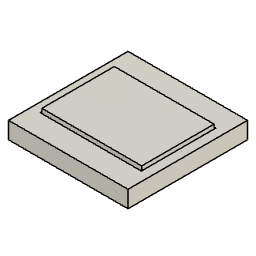
EU_switch (Autodesk Fusion 360 design; units mm, degrees)
Autodesk Fusion 360 part; units mm, degrees
note: some values were not read from the file. Set by a fixed rule: which sketch regions a step uses.
box "BoxPrimitive3" add length 85 width 85 height 12 placed x (0, 1, 0) y (-1, 0, 0) z (0, 0, 1) at (85, 0, 0) makes body 1 in component "panel"
ref_plane "WorkPlane1" through (42.5, 42.5, 12) normal (0, 0, 1) x (0, 1, 0) in component "panel"
sketch "Sketch5" plane through (42.5, 42.5, 12) normal (0, 0, 1) x (1, 0, 0) in component "panel"
  line L0 (-36, 26.5) -> (36, 26.5)
  line L1 (36, 26.5) -> (36, -26.5)
  line L2 (36, -26.5) -> (-36, -26.5)
  line L3 (-36, -26.5) -> (-36, 26.5)
  dimension "d59" = 72
  dimension "d60" = 53
  dimension "d61" = 36
  dimension "d63" = 26.5
  constraint horizontal L0
  constraint vertical L1
  constraint horizontal L2
  constraint vertical L3
  measures "d59" distance of L0.start L0.end
  measures "d60" distance of L0.start L2.end
  measures "d61" distance of origin L1
  measures "d63" distance of origin L0
extrude "Extrude3" cut sketch "Sketch5" against normal through all bodies 1 in component "panel"
ref_plane "WorkPlane2" through (42.5, 42.5, 0) normal (0, 0, -1) x (0, -1, 0) in component "panel"
sketch "Sketch7" plane through (42.5, 42.5, 0) normal (0, 0, -1) x (1, 0, 0) in component "panel"
  line L0 (-40, 40) -> (40, 40)
  line L1 (40, 40) -> (40, -40)
  line L2 (40, -40) -> (-40, -40)
  line L3 (-40, -40) -> (-40, 40)
  line L4 (-42.5, 42.5) -> (-42.5, -42.5)
  line L5 (42.5, -42.5) -> (42.5, 42.5)
  line L6 (42.5, 42.5) -> (-42.5, 42.5)
  line L7 (-42.5, -42.5) -> (42.5, -42.5)
  dimension "d110" = 2.5
  dimension "d112" = 2.5
  dimension "d113" = 2.5
  dimension "d114" = 2.5
  constraint horizontal L0
  constraint vertical L1
  constraint horizontal L2
  constraint vertical L3
  measures "d110" distance of L0.start L4
  measures "d112" distance of L0.end L5
  measures "d113" distance of L0.start L6
  measures "d114" distance of L2.end L7
extrude "Extrude4" cut sketch "Sketch7" against normal blind 10 contours L0 L1 L2 L3 bodies 1 in component "panel"
ref_plane "WorkPlane1" through (42.5, 42.5, 11) normal (-1, 0, 0) x (0, 1, 0) in component "Button"
sketch "Sketch3" plane through (42.5, 42.5, 11) normal (-1, 0, 0) x (0, 1, 0) in component "Button"
  line L0 (-25.7589, 3.5328) -> (-25.7589, -3.5328)
  line L1 (-25.7589, -3.5328) -> (25.7589, -3.5328)
  line L2 (25.7589, -3.5328) -> (25.7589, 3.5328)
  line L3 (25.7589, 3.5328) -> (-25.7589, 3.5328)
  line L4 (-25.7589, 3.5328) -> (25.7589, -3.5328) construction
  line L5 (-25.7589, -3.5328) -> (25.7589, 3.5328) construction
  line L6 (-25.7589, -3.5328) -> (-24.8077, 3.4023) construction
  line L7 (25.7589, -3.5328) -> (24.8077, 3.4023) construction
  line L8 (0, 0) -> (0, -3.5328) construction
  dimension "d96" = 7
  dimension "d97" = 52
  constraint perpendicular L0 L1
  constraint perpendicular L1 L2
  constraint coincident L0 L3.end
  constraint perpendicular L0 L3
  constraint coincident L4 L6.end
  constraint coincident L5 L7.end
  constraint perpendicular L5 L7
  constraint perpendicular L4 L6
  constraint midpoint L4 L8.start
  constraint midpoint L1 L8.end
  constraint coincident L8.start origin
  measures "d96" distance of L0.end L6.end
  measures "d97" distance of L1.end L0.start
extrude "Extrude1" add sketch "Sketch3" along normal mid plane 71 separate body makes body 2 in component "Button"
ref_plane "WorkPlane4" through (42.5, 42.5, 11) normal (1, 0, 0) x (0, -1, 0) in component "panel"
sketch "Sketch9" plane through (42.5, 42.5, 11) normal (1, 0, 0) x (0, 1, 0) in component "panel"
  circle A0 centre (0, 0) radius 0.5
  dimension "d100" = 1
  constraint coincident A0.centre origin
  measures "d100" diameter of A0
extrude "Extrude6" cut sketch "Sketch9" along normal mid plane 76 bodies 1 in component "panel"
sketch "Sketch4" plane through (42.5, 42.5, 11) normal (-1, 0, 0) x (0, 1, 0) in component "Button"
  circle A0 centre (0, 0) radius 0.5
  dimension "d103" = 1
  constraint coincident A0.centre origin
  measures "d103" diameter of A0
extrude "Extrude2" add sketch "Sketch4" along normal mid plane 76 bodies 2 in component "Button"
component "panel" placed x (1, 0, 0) y (0, 1, 0) z (0, 0, 1) at (0, 0, 0)
component "Button" placed x (1, 0, 0) y (0, 1, 0) z (0, 0, 1) at (0, 0, 0)
named bodies: "Body1"
